Autodesk Fusion 360 part; units mm, degrees
(part 3 of 7)
  line L362 (75.7834, -59.8105) -> (75.8535, -59.6632)
  line L363 (75.8535, -59.6632) -> (76.1212, -59.7821)
  line L364 (76.1212, -59.7821) -> (76.1988, -59.8037)
  line L365 (76.1988, -59.8037) -> (76.2804, -59.8161)
  line L366 (76.2804, -59.8161) -> (76.3647, -59.822)
  line L367 (76.3647, -59.822) -> (76.451, -59.8224)
  line L368 (76.451, -59.8224) -> (76.5391, -59.8175)
  line L369 (76.5391, -59.8175) -> (76.6286, -59.8079)
  line L370 (76.6286, -59.8079) -> (76.7195, -59.7936)
  line L371 (76.7195, -59.7936) -> (76.8114, -59.7747)
  line L372 (76.8114, -59.7747) -> (76.9043, -59.7514)
  line L373 (76.9043, -59.7514) -> (76.9979, -59.7237)
  line L374 (76.9979, -59.7237) -> (77.0921, -59.6916)
  line L375 (77.0921, -59.6916) -> (77.1867, -59.6553)
  line L376 (77.1867, -59.6553) -> (77.2104, -59.5733)
  line L377 (77.2104, -59.5733) -> (77.2325, -59.4909)
  line L378 (77.2325, -59.4909) -> (77.2529, -59.4081)
  line L379 (77.2529, -59.4081) -> (77.1891, -59.3293)
  line L380 (77.1891, -59.3293) -> (77.1236, -59.2545)
  line L381 (77.1236, -59.2545) -> (77.0564, -59.1837)
  line L382 (77.0564, -59.1837) -> (76.9876, -59.117)
  line L383 (76.9876, -59.117) -> (76.9175, -59.0547)
  line L384 (76.9175, -59.0547) -> (76.8459, -58.9969)
  line L385 (76.8459, -58.9969) -> (76.7732, -58.9437)
  line L386 (76.7732, -58.9437) -> (76.6993, -58.8955)
  line L387 (76.6993, -58.8955) -> (76.6244, -58.8526)
  line L388 (76.6244, -58.8526) -> (76.5485, -58.8156)
  line L389 (76.5485, -58.8156) -> (76.4716, -58.7856)
  line L390 (76.4716, -58.7856) -> (76.3936, -58.7655)
  line L391 (76.3936, -58.7655) -> (76.1023, -58.7347)
  line L392 (76.1023, -58.7347) -> (76.1152, -58.572)
  line L393 (76.1152, -58.572) -> (76.1195, -58.4089)
  line L394 (76.1195, -58.4089) -> (76.1152, -58.2458)
  line L395 (76.1152, -58.2458) -> (76.1023, -58.0831)
extrude "Extrude2" add sketch "Sketch2" along normal blind 2.3 separate body makes body 3 in component "CT idler 1"
combine "Combine1" operation add target body 2 tool bodies 3 in component "CT idler 1"
ref_plane "WorkPlane3" through (0, 0, 36.8) normal (0, 0, 1) x (1, 0, 0) in component "CT idler 1"
sketch "Sketch3" plane through (0, 0, 36.8) normal (0, 0, 1) x (1, 0, 0) in component "CT idler 1"
  circle A0 centre (73.0295, -58.4089) radius 2.1
extrude "Extrude3" cut sketch "Sketch3" along normal blind 2 bodies 2 in component "CT idler 1"
ref_plane "WorkPlane4" through (0, 0, 38.8) normal (0, 0, 1) x (1, 0, 0) in component "CT idler 1"
sketch "Sketch4" plane through (0, 0, 38.8) normal (0, 0, 1) x (1, 0, 0) in component "CT idler 1"
  circle A0 centre (73.0295, -58.4089) radius 1.7
extrude "Extrude4" cut sketch "Sketch4" along normal blind 2 bodies 2 in component "CT idler 1"
ref_plane "WorkPlane1" through (0, 0, 39) normal (0, 0, 1) x (1, 0, 0) in component "CT idler 2"
sketch "Sketch1 (3)" plane through (0, 0, 39) normal (0, 0, 1) x (1, 0, 0) in component "CT idler 2"
  line L0 (65.785, -68.2435) -> (66.0567, -68.5986)
  line L1 (66.0567, -68.5986) -> (66.1054, -68.6519)
  line L2 (66.1054, -68.6519) -> (66.1583, -68.702)
  line L3 (66.1583, -68.702) -> (66.2139, -68.7499)
  line L4 (66.2139, -68.7499) -> (66.2719, -68.796)
  line L5 (66.2719, -68.796) -> (66.3318, -68.8405)
  line L6 (66.3318, -68.8405) -> (66.3935, -68.8835)
  line L7 (66.3935, -68.8835) -> (66.457, -68.9251)
  line L8 (66.457, -68.9251) -> (66.522, -68.9654)
  line L9 (66.522, -68.9654) -> (66.5885, -69.0044)
  line L10 (66.5885, -69.0044) -> (66.6564, -69.0422)
  line L11 (66.6564, -69.0422) -> (66.7256, -69.0788)
  line L12 (66.7256, -69.0788) -> (66.7962, -69.1142)
  line L13 (66.7962, -69.1142) -> (66.9045, -69.0248)
  line L14 (66.9045, -69.0248) -> (67.0114, -68.9338)
  line L15 (67.0114, -68.9338) -> (67.117, -68.8411)
  line L16 (67.117, -68.8411) -> (67.0933, -68.7658)
  line L17 (67.0933, -68.7658) -> (67.0683, -68.6916)
  line L18 (67.0683, -68.6916) -> (67.0418, -68.6186)
  line L19 (67.0418, -68.6186) -> (67.014, -68.5467)
  line L20 (67.014, -68.5467) -> (66.9846, -68.4761)
  line L21 (66.9846, -68.4761) -> (66.9536, -68.4068)
  line L22 (66.9536, -68.4068) -> (66.921, -68.339)
  line L23 (66.921, -68.339) -> (66.8867, -68.2727)
  line L24 (66.8867, -68.2727) -> (66.8505, -68.2082)
  line L25 (66.8505, -68.2082) -> (66.8121, -68.1456)
  line L26 (66.8121, -68.1456) -> (66.7711, -68.0854)
  line L27 (66.7711, -68.0854) -> (66.7263, -68.0288)
  line L28 (66.7263, -68.0288) -> (66.4191, -67.7038)
  line L29 (66.4191, -67.7038) -> (66.5706, -67.5567)
  line L30 (66.5706, -67.5567) -> (66.7182, -67.4058)
  line L31 (66.7182, -67.4058) -> (66.8618, -67.251)
  line L32 (66.8618, -67.251) -> (67.0012, -67.0925)
  line L33 (67.0012, -67.0925) -> (67.3409, -67.3834)
  line L34 (67.3409, -67.3834) -> (67.3996, -67.4254)
  line L35 (67.3996, -67.4254) -> (67.4617, -67.4634)
  line L36 (67.4617, -67.4634) -> (67.5261, -67.4986)
  line L37 (67.5261, -67.4986) -> (67.5924, -67.5317)
  line L38 (67.5924, -67.5317) -> (67.6602, -67.5627)
  line L39 (67.6602, -67.5627) -> (67.7296, -67.592)
  line L40 (67.7296, -67.592) -> (67.8003, -67.6195)
  line L41 (67.8003, -67.6195) -> (67.8722, -67.6454)
  line L42 (67.8722, -67.6454) -> (67.9454, -67.6698)
  line L43 (67.9454, -67.6698) -> (68.0197, -67.6926)
  line L44 (68.0197, -67.6926) -> (68.095, -67.714)
  line L45 (68.095, -67.714) -> (68.1714, -67.7339)
  line L46 (68.1714, -67.7339) -> (68.2587, -67.624)
  line L47 (68.2587, -67.624) -> (68.3444, -67.5127)
  line L48 (68.3444, -67.5127) -> (68.4284, -67.4001)
  line L49 (68.4284, -67.4001) -> (68.3896, -67.3314)
  line L50 (68.3896, -67.3314) -> (68.3497, -67.264)
  line L51 (68.3497, -67.264) -> (68.3086, -67.1981)
  line L52 (68.3086, -67.1981) -> (68.2664, -67.1336)
  line L53 (68.2664, -67.1336) -> (68.223, -67.0706)
  line L54 (68.223, -67.0706) -> (68.1783, -67.0093)
  line L55 (68.1783, -67.0093) -> (68.1323, -66.9497)
  line L56 (68.1323, -66.9497) -> (68.085, -66.892)
  line L57 (68.085, -66.892) -> (68.0361, -66.8364)
  line L58 (68.0361, -66.8364) -> (67.9855, -66.7832)
  line L59 (67.9855, -66.7832) -> (67.933, -66.7328)
  line L60 (67.933, -66.7328) -> (67.8774, -66.6868)
  line L61 (67.8774, -66.6868) -> (67.5093, -66.4327)
  line L62 (67.5093, -66.4327) -> (67.627, -66.2574)
  line L63 (67.627, -66.2574) -> (67.74, -66.0791)
  line L64 (67.74, -66.0791) -> (67.8482, -65.8978)
  line L65 (67.8482, -65.8978) -> (67.9516, -65.7137)
  line L66 (67.9516, -65.7137) -> (68.3444, -65.9277)
  line L67 (68.3444, -65.9277) -> (68.4105, -65.9566)
  line L68 (68.4105, -65.9566) -> (68.4792, -65.9808)
  line L69 (68.4792, -65.9808) -> (68.5495, -66.0019)
  line L70 (68.5495, -66.0019) -> (68.6212, -66.0205)
  line L71 (68.6212, -66.0205) -> (68.694, -66.0367)
  line L72 (68.694, -66.0367) -> (68.7679, -66.0509)
  line L73 (68.7679, -66.0509) -> (68.8428, -66.0631)
  line L74 (68.8428, -66.0631) -> (68.9186, -66.0735)
  line L75 (68.9186, -66.0735) -> (68.9952, -66.0821)
  line L76 (68.9952, -66.0821) -> (69.0726, -66.089)
  line L77 (69.0726, -66.089) -> (69.1507, -66.0943)
  line L78 (69.1507, -66.0943) -> (69.2295, -66.0979)
  line L79 (69.2295, -66.0979) -> (69.2921, -65.9722)
  line L80 (69.2921, -65.9722) -> (69.3528, -65.8455)
  line L81 (69.3528, -65.8455) -> (69.4116, -65.718)
  line L82 (69.4116, -65.718) -> (69.3593, -65.6588)
  line L83 (69.3593, -65.6588) -> (69.3063, -65.6012)
  line L84 (69.3063, -65.6012) -> (69.2524, -65.5452)
  line L85 (69.2524, -65.5452) -> (69.1977, -65.4909)
  line L86 (69.1977, -65.4909) -> (69.1421, -65.4383)
  line L87 (69.1421, -65.4383) -> (69.0857, -65.3877)
  line L88 (69.0857, -65.3877) -> (69.0283, -65.3389)
  line L89 (69.0283, -65.3389) -> (68.97, -65.2924)
  line L90 (68.97, -65.2924) -> (68.9106, -65.2481)
  line L91 (68.9106, -65.2481) -> (68.8501, -65.2066)
  line L92 (68.8501, -65.2066) -> (68.7882, -65.1682)
  line L93 (68.7882, -65.1682) -> (68.7243, -65.1348)
  line L94 (68.7243, -65.1348) -> (68.3114, -64.9628)
  line L95 (68.3114, -64.9628) -> (68.3901, -64.7668)
  line L96 (68.3901, -64.7668) -> (68.4635, -64.5689)
  line L97 (68.4635, -64.5689) -> (68.5317, -64.3691)
  line L98 (68.5317, -64.3691) -> (68.5946, -64.1676)
  line L99 (68.5946, -64.1676) -> (69.0232, -64.2952)
  line L100 (69.0232, -64.2952) -> (69.0939, -64.3097)
  line L101 (69.0939, -64.3097) -> (69.1661, -64.3191)
  line L102 (69.1661, -64.3191) -> (69.2393, -64.3251)
  line L103 (69.2393, -64.3251) -> (69.3133, -64.3284)
  line L104 (69.3133, -64.3284) -> (69.3879, -64.3291)
  line L105 (69.3879, -64.3291) -> (69.4631, -64.3276)
  line L106 (69.4631, -64.3276) -> (69.5389, -64.324)
  line L107 (69.5389, -64.324) -> (69.6152, -64.3184)
  line L108 (69.6152, -64.3184) -> (69.6919, -64.3109)
  line L109 (69.6919, -64.3109) -> (69.7691, -64.3016)
  line L110 (69.7691, -64.3016) -> (69.8466, -64.2905)
  line L111 (69.8466, -64.2905) -> (69.9245, -64.2776)
  line L112 (69.9245, -64.2776) -> (69.9595, -64.1416)
  line L113 (69.9595, -64.1416) -> (69.9926, -64.0051)
  line L114 (69.9926, -64.0051) -> (70.0235, -63.8682)
  line L115 (70.0235, -63.8682) -> (69.9601, -63.8211)
  line L116 (69.9601, -63.8211) -> (69.8963, -63.7758)
  line L117 (69.8963, -63.7758) -> (69.8319, -63.7323)
  line L118 (69.8319, -63.7323) -> (69.7671, -63.6905)
  line L119 (69.7671, -63.6905) -> (69.7018, -63.6507)
  line L120 (69.7018, -63.6507) -> (69.6361, -63.6128)
  line L121 (69.6361, -63.6128) -> (69.5698, -63.5771)
  line L122 (69.5698, -63.5771) -> (69.5031, -63.5436)
  line L123 (69.5031, -63.5436) -> (69.4358, -63.5127)
  line L124 (69.4358, -63.5127) -> (69.368, -63.4847)
  line L125 (69.368, -63.4847) -> (69.2995, -63.46)
  line L126 (69.2995, -63.46) -> (69.23, -63.4406)
  line L127 (69.23, -63.4406) -> (68.7904, -63.3582)
  line L128 (68.7904, -63.3582) -> (68.8266, -63.1502)
  line L129 (68.8266, -63.1502) -> (68.8573, -62.9413)
  line L130 (68.8573, -62.9413) -> (68.8824, -62.7317)
  line L131 (68.8824, -62.7317) -> (68.9021, -62.5215)
  line L132 (68.9021, -62.5215) -> (69.3479, -62.5572)
  line L133 (69.3479, -62.5572) -> (69.42, -62.5567)
  line L134 (69.42, -62.5567) -> (69.4926, -62.5509)
  line L135 (69.4926, -62.5509) -> (69.5654, -62.5416)
  line L136 (69.5654, -62.5416) -> (69.6384, -62.5294)
  line L137 (69.6384, -62.5294) -> (69.7116, -62.5146)
  line L138 (69.7116, -62.5146) -> (69.7849, -62.4975)
  line L139 (69.7849, -62.4975) -> (69.8583, -62.4782)
  line L140 (69.8583, -62.4782) -> (69.9317, -62.4569)
  line L141 (69.9317, -62.4569) -> (70.0052, -62.4336)
  line L142 (70.0052, -62.4336) -> (70.0787, -62.4084)
  line L143 (70.0787, -62.4084) -> (70.1522, -62.3814)
  line L144 (70.1522, -62.3814) -> (70.2257, -62.3526)
  line L145 (70.2257, -62.3526) -> (70.2318, -62.2123)
  line L146 (70.2318, -62.2123) -> (70.2357, -62.072)
  line L147 (70.2357, -62.072) -> (70.2375, -61.9315)
  line L148 (70.2375, -61.9315) -> (70.1657, -61.8987)
  line L149 (70.1657, -61.8987) -> (70.0938, -61.8677)
  line L150 (70.0938, -61.8677) -> (70.0218, -61.8384)
  line L151 (70.0218, -61.8384) -> (69.9498, -61.8111)
  line L152 (69.9498, -61.8111) -> (69.8776, -61.7857)
  line L153 (69.8776, -61.7857) -> (69.8054, -61.7623)
  line L154 (69.8054, -61.7623) -> (69.7332, -61.7411)
  line L155 (69.7332, -61.7411) -> (69.661, -61.7223)
  line L156 (69.661, -61.7223) -> (69.5888, -61.706)
  line L157 (69.5888, -61.706) -> (69.5166, -61.6927)
  line L158 (69.5166, -61.6927) -> (69.4444, -61.6829)
  line L159 (69.4444, -61.6829) -> (69.3724, -61.6783)
  line L160 (69.3724, -61.6783) -> (68.9253, -61.6891)
  line L161 (68.9253, -61.6891) -> (68.9174, -61.4781)
  line L162 (68.9174, -61.4781) -> (68.904, -61.2674)
  line L163 (68.904, -61.2674) -> (68.885, -61.0571)
  line L164 (68.885, -61.0571) -> (68.8605, -60.8474)
  line L165 (68.8605, -60.8474) -> (69.304, -60.7897)
  line L166 (69.304, -60.7897) -> (69.3745, -60.7742)
  line L167 (69.3745, -60.7742) -> (69.4443, -60.7534)
  line L168 (69.4443, -60.7534) -> (69.5136, -60.7292)
  line L169 (69.5136, -60.7292) -> (69.5825, -60.7021)
  line L170 (69.5825, -60.7021) -> (69.651, -60.6724)
  line L171 (69.651, -60.6724) -> (69.7191, -60.6404)
  line L172 (69.7191, -60.6404) -> (69.7869, -60.6063)
  line L173 (69.7869, -60.6063) -> (69.8543, -60.5702)
  line L174 (69.8543, -60.5702) -> (69.9213, -60.5321)
  line L175 (69.9213, -60.5321) -> (69.988, -60.4922)
  line L176 (69.988, -60.4922) -> (70.0543, -60.4505)
  line L177 (70.0543, -60.4505) -> (70.1202, -60.4071)
  line L178 (70.1202, -60.4071) -> (70.0969, -60.2686)
  line L179 (70.0969, -60.2686) -> (70.0716, -60.1305)
  line L180 (70.0716, -60.1305) -> (70.0441, -59.9928)
  line L181 (70.0441, -59.9928) -> (69.9671, -59.9756)
  line L182 (69.9671, -59.9756) -> (69.8903, -59.9602)
  line L183 (69.8903, -59.9602) -> (69.8138, -59.9465)
  line L184 (69.8138, -59.9465) -> (69.7377, -59.9347)
  line L185 (69.7377, -59.9347) -> (69.6618, -59.9249)
  line L186 (69.6618, -59.9249) -> (69.5863, -59.9171)
  line L187 (69.5863, -59.9171) -> (69.5113, -59.9114)
  line L188 (69.5113, -59.9114) -> (69.4367, -59.908)
  line L189 (69.4367, -59.908) -> (69.3627, -59.9071)
  line L190 (69.3627, -59.9071) -> (69.2893, -59.909)
  line L191 (69.2893, -59.909) -> (69.2167, -59.9144)
  line L192 (69.2167, -59.9144) -> (69.1453, -59.9249)
  line L193 (69.1453, -59.9249) -> (68.7102, -60.0284)
  line L194 (68.7102, -60.0284) -> (68.6587, -59.8237)
  line L195 (68.6587, -59.8237) -> (68.6017, -59.6204)
  line L196 (68.6017, -59.6204) -> (68.5395, -59.4186)
  line L197 (68.5395, -59.4186) -> (68.4719, -59.2186)
  line L198 (68.4719, -59.2186) -> (68.8937, -59.0699)
  line L199 (68.8937, -59.0699) -> (68.9594, -59.0401)
  line L200 (68.9594, -59.0401) -> (69.0233, -59.0053)
  line L201 (69.0233, -59.0053) -> (69.0861, -58.9672)
  line L202 (69.0861, -58.9672) -> (69.1478, -58.9263)
  line L203 (69.1478, -58.9263) -> (69.2087, -58.8831)
  line L204 (69.2087, -58.8831) -> (69.2687, -58.8376)
  line L205 (69.2687, -58.8376) -> (69.3278, -58.7902)
  line L206 (69.3278, -58.7902) -> (69.3863, -58.7408)
  line L207 (69.3863, -58.7408) -> (69.4439, -58.6896)
  line L208 (69.4439, -58.6896) -> (69.5008, -58.6367)
  line L209 (69.5008, -58.6367) -> (69.557, -58.5822)
  line L210 (69.557, -58.5822) -> (69.6125, -58.526)
  line L211 (69.6125, -58.526) -> (69.5609, -58.3954)
  line L212 (69.5609, -58.3954) -> (69.5074, -58.2655)
  line L213 (69.5074, -58.2655) -> (69.4519, -58.1365)
  line L214 (69.4519, -58.1365) -> (69.373, -58.1357)
  line L215 (69.373, -58.1357) -> (69.2947, -58.1366)
  line L216 (69.2947, -58.1366) -> (69.217, -58.1392)
  line L217 (69.217, -58.1392) -> (69.1401, -58.1435)
  line L218 (69.1401, -58.1435) -> (69.0638, -58.1496)
  line L219 (69.0638, -58.1496) -> (68.9884, -58.1577)
  line L220 (68.9884, -58.1577) -> (68.9138, -58.1677)
  line L221 (68.9138, -58.1677) -> (68.8402, -58.1799)
  line L222 (68.8402, -58.1799) -> (68.7676, -58.1944)
  line L223 (68.7676, -58.1944) -> (68.6962, -58.2115)
  line L224 (68.6962, -58.2115) -> (68.6263, -58.2319)
  line L225 (68.6263, -58.2319) -> (68.5586, -58.2571)
  line L226 (68.5586, -58.2571) -> (68.1546, -58.4487)
  line L227 (68.1546, -58.4487) -> (68.0616, -58.2592)
  line L228 (68.0616, -58.2592) -> (67.9636, -58.0722)
  line L229 (67.9636, -58.0722) -> (67.8608, -57.8878)
  line L230 (67.8608, -57.8878) -> (67.7531, -57.7062)
  line L231 (67.7531, -57.7062) -> (68.1347, -57.4731)
  line L232 (68.1347, -57.4731) -> (68.1928, -57.4302)
  line L233 (68.1928, -57.4302) -> (68.2481, -57.3829)
  line L234 (68.2481, -57.3829) -> (68.3016, -57.3325)
  line L235 (68.3016, -57.3325) -> (68.3535, -57.2797)
  line L236 (68.3535, -57.2797) -> (68.404, -57.2248)
  line L237 (68.404, -57.2248) -> (68.4532, -57.1679)
  line L238 (68.4532, -57.1679) -> (68.5012, -57.1091)
  line L239 (68.5012, -57.1091) -> (68.5481, -57.0487)
  line L240 (68.5481, -57.0487) -> (68.5939, -56.9867)
  line L241 (68.5939, -56.9867) -> (68.6385, -56.9231)
  line L242 (68.6385, -56.9231) -> (68.6822, -56.858)
  line L243 (68.6822, -56.858) -> (68.7247, -56.7916)
  line L244 (68.7247, -56.7916) -> (68.6471, -56.6745)
  line L245 (68.6471, -56.6745) -> (68.5678, -56.5587)
  line L246 (68.5678, -56.5587) -> (68.4867, -56.444)
  line L247 (68.4867, -56.444) -> (68.4094, -56.4596)
  line L248 (68.4094, -56.4596) -> (68.3329, -56.4768)
  line L249 (68.3329, -56.4768) -> (68.2575, -56.4954)
  line L250 (68.2575, -56.4954) -> (68.1831, -56.5157)
  line L251 (68.1831, -56.5157) -> (68.1098, -56.5375)
  line L252 (68.1098, -56.5375) -> (68.0377, -56.561)
  line L253 (68.0377, -56.561) -> (67.9668, -56.5864)
  line L254 (67.9668, -56.5864) -> (67.8973, -56.6136)
  line L255 (67.8973, -56.6136) -> (67.8293, -56.6429)
  line L256 (67.8293, -56.6429) -> (67.7631, -56.6745)
  line L257 (67.7631, -56.6745) -> (67.6989, -56.709)
  line L258 (67.6989, -56.709) -> (67.638, -56.7476)
  line L259 (67.638, -56.7476) -> (67.2826, -57.0191)
  line L260 (67.2826, -57.0191) -> (67.1522, -56.8531)
  line L261 (67.1522, -56.8531) -> (67.0175, -56.6905)
  line L262 (67.0175, -56.6905) -> (66.8786, -56.5315)
  line L263 (66.8786, -56.5315) -> (66.7355, -56.3763)
  line L264 (66.7355, -56.3763) -> (67.0604, -56.0689)
  line L265 (67.0604, -56.0689) -> (67.1083, -56.0149)
  line L266 (67.1083, -56.0149) -> (67.1525, -55.9571)
  line L267 (67.1525, -55.9571) -> (67.1943, -55.8967)
  line L268 (67.1943, -55.8967) -> (67.2341, -55.8343)
  line L269 (67.2341, -55.8343) -> (67.2721, -55.7701)
  line L270 (67.2721, -55.7701) -> (67.3084, -55.7041)
  line L271 (67.3084, -55.7041) -> (67.3432, -55.6367)
  line L272 (67.3432, -55.6367) -> (67.3765, -55.5679)
  line L273 (67.3765, -55.5679) -> (67.4083, -55.4977)
  line L274 (67.4083, -55.4977) -> (67.4388, -55.4262)
  line L275 (67.4388, -55.4262) -> (67.468, -55.3535)
  line L276 (67.468, -55.3535) -> (67.4958, -55.2796)
  line L277 (67.4958, -55.2796) -> (67.3955, -55.1813)
  line L278 (67.3955, -55.1813) -> (67.2938, -55.0844)
  line L279 (67.2938, -55.0844) -> (67.1907, -54.9891)
  line L280 (67.1907, -54.9891) -> (67.1183, -55.0205)
  line L281 (67.1183, -55.0205) -> (67.0471, -55.0532)
  line L282 (67.0471, -55.0532) -> (66.9772, -55.0871)
  line L283 (66.9772, -55.0871) -> (66.9086, -55.1223)
  line L284 (66.9086, -55.1223) -> (66.8415, -55.1589)
  line L285 (66.8415, -55.1589) -> (66.7758, -55.197)
  line L286 (66.7758, -55.197) -> (66.7118, -55.2365)
  line L287 (66.7118, -55.2365) -> (66.6495, -55.2775)
  line L288 (66.6495, -55.2775) -> (66.589, -55.3203)
  line L289 (66.589, -55.3203) -> (66.5308, -55.365)
  line L290 (66.5308, -55.365) -> (66.4752, -55.4121)
  line L291 (66.4752, -55.4121) -> (66.4237, -55.4626)
  line L292 (66.4237, -55.4626) -> (66.1325, -55.802)
  line L293 (66.1325, -55.802) -> (65.9704, -55.6667)
  line L294 (65.9704, -55.6667) -> (65.8049, -55.5357)
  line L295 (65.8049, -55.5357) -> (65.6359, -55.4091)
  line L296 (65.6359, -55.4091) -> (65.4637, -55.287)
  line L297 (65.4637, -55.287) -> (65.7175, -54.9188)
  line L298 (65.7175, -54.9188) -> (65.7532, -54.856)
  line L299 (65.7532, -54.856) -> (65.7844, -54.7903)
  line L300 (65.7844, -54.7903) -> (65.8128, -54.7225)
  line L301 (65.8128, -54.7225) -> (65.8387, -54.6532)
  line L302 (65.8387, -54.6532) -> (65.8625, -54.5824)
  line L303 (65.8625, -54.5824) -> (65.8844, -54.5104)
  line L304 (65.8844, -54.5104) -> (65.9043, -54.4372)
  line L305 (65.9043, -54.4372) -> (65.9226, -54.363)
  line L306 (65.9226, -54.363) -> (65.9391, -54.2877)
  line L307 (65.9391, -54.2877) -> (65.9541, -54.2114)
  line L308 (65.9541, -54.2114) -> (65.9675, -54.1343)
  line L309 (65.9675, -54.1343) -> (65.9793, -54.0562)
  line L310 (65.9793, -54.0562) -> (65.8608, -53.9809)
  line L311 (65.8608, -53.9809) -> (65.7412, -53.9073)
  line L312 (65.7412, -53.9073) -> (65.6205, -53.8355)
  line L313 (65.6205, -53.8355) -> (65.5562, -53.8813)
  line L314 (65.5562, -53.8813) -> (65.4934, -53.928)
  line L315 (65.4934, -53.928) -> (65.4321, -53.9757)
  line L316 (65.4321, -53.9757) -> (65.3723, -54.0244)
  line L317 (65.3723, -54.0244) -> (65.3143, -54.0742)
  line L318 (65.3143, -54.0742) -> (65.2579, -54.1251)
  line L319 (65.2579, -54.1251) -> (65.2035, -54.177)
  line L320 (65.2035, -54.177) -> (65.1511, -54.2301)
  line L321 (65.1511, -54.2301) -> (65.1009, -54.2846)
  line L322 (65.1009, -54.2846) -> (65.0532, -54.3404)
  line L323 (65.0532, -54.3404) -> (65.0086, -54.398)
  line L324 (65.0086, -54.398) -> (64.9687, -54.4581)
  line L325 (64.9687, -54.4581) -> (64.7545, -54.8507)
  line L326 (64.7545, -54.8507) -> (64.5678, -54.752)
  line L327 (64.5678, -54.752) -> (64.3786, -54.6583)
  line L328 (64.3786, -54.6583) -> (64.187, -54.5695)
  line L329 (64.187, -54.5695) -> (63.9932, -54.4859)
  line L330 (63.9932, -54.4859) -> (64.1649, -54.073)
  line L331 (64.1649, -54.073) -> (64.1867, -54.0042)
  line L332 (64.1867, -54.0042) -> (64.2036, -53.9334)
  line L333 (64.2036, -53.9334) -> (64.2173, -53.8612)
  line L334 (64.2173, -53.8612) -> (64.2283, -53.788)
  line L335 (64.2283, -53.788) -> (64.2368, -53.7139)
  line L336 (64.2368, -53.7139) -> (64.2432, -53.6389)
  line L337 (64.2432, -53.6389) -> (64.2475, -53.5631)
  line L338 (64.2475, -53.5631) -> (64.2499, -53.4867)
  line L339 (64.2499, -53.4867) -> (64.2505, -53.4096)
  line L340 (64.2505, -53.4096) -> (64.2492, -53.3319)
  line L341 (64.2492, -53.3319) -> (64.2463, -53.2536)
  line L342 (64.2463, -53.2536) -> (64.2417, -53.1749)
  line L343 (64.2417, -53.1749) -> (64.1101, -53.1258)
  line L344 (64.1101, -53.1258) -> (63.9778, -53.0786)
  line L345 (63.9778, -53.0786) -> (63.8448, -53.0335)
  line L346 (63.8448, -53.0335) -> (63.7914, -53.0917)
  line L347 (63.7914, -53.0917) -> (63.7397, -53.1504)
  line L348 (63.7397, -53.1504) -> (63.6896, -53.2099)
  line L349 (63.6896, -53.2099) -> (63.6413, -53.27)
  line L350 (63.6413, -53.27) -> (63.5949, -53.3307)
  line L351 (63.5949, -53.3307) -> (63.5503, -53.3922)
  line L352 (63.5503, -53.3922) -> (63.5079, -53.4543)
  line L353 (63.5079, -53.4543) -> (63.4677, -53.5172)
  line L354 (63.4677, -53.5172) -> (63.4299, -53.5808)
  line L355 (63.4299, -53.5808) -> (63.3949, -53.6454)
  line L356 (63.3949, -53.6454) -> (63.3632, -53.7109)
  line L357 (63.3632, -53.7109) -> (63.3367, -53.778)
  line L358 (63.3367, -53.778) -> (63.2087, -54.2066)
  line L359 (63.2087, -54.2066) -> (63.0056, -54.1489)
  line L360 (63.0056, -54.1489) -> (62.8011, -54.0965)
  line L361 (62.8011, -54.0965) -> (62.5953, -54.0496)
  line L362 (62.5953, -54.0496) -> (62.3883, -54.0081)
  line L363 (62.3883, -54.0081) -> (62.4704, -53.5685)
  line L364 (62.4704, -53.5685) -> (62.4774, -53.4966)
  line L365 (62.4774, -53.4966) -> (62.4792, -53.4239)
  line L366 (62.4792, -53.4239) -> (62.4776, -53.3505)
  line L367 (62.4776, -53.3505) -> (62.4731, -53.2766)
  line L368 (62.4731, -53.2766) -> (62.466, -53.2022)
  line L369 (62.466, -53.2022) -> (62.4567, -53.1276)
  line L370 (62.4567, -53.1276) -> (62.4452, -53.0526)
  line L371 (62.4452, -53.0526) -> (62.4316, -52.9773)
  line L372 (62.4316, -52.9773) -> (62.4161, -52.9018)
  line L373 (62.4161, -52.9018) -> (62.3988, -52.8261)
  line L374 (62.3988, -52.8261) -> (62.3796, -52.7501)
  line L375 (62.3796, -52.7501) -> (62.3587, -52.674)
  line L376 (62.3587, -52.674) -> (62.2198, -52.6533)
  line L377 (62.2198, -52.6533) -> (62.0806, -52.6348)
  line L378 (62.0806, -52.6348) -> (61.9412, -52.6183)
  line L379 (61.9412, -52.6183) -> (61.901, -52.6863)
  line L380 (61.901, -52.6863) -> (61.8626, -52.7545)
  line L381 (61.8626, -52.7545) -> (61.826, -52.8231)
  line L382 (61.826, -52.8231) -> (61.7913, -52.8919)
  line L383 (61.7913, -52.8919) -> (61.7585, -52.961)
  line L384 (61.7585, -52.961) -> (61.7277, -53.0303)
  line L385 (61.7277, -53.0303) -> (61.6991, -53.0999)
  line L386 (61.6991, -53.0999) -> (61.6728, -53.1698)
  line L387 (61.6728, -53.1698) -> (61.6491, -53.2399)
  line L388 (61.6491, -53.2399) -> (61.6283, -53.3103)
  line L389 (61.6283, -53.3103) -> (61.6109, -53.381)
  line L390 (61.6109, -53.381) -> (61.5989, -53.4522)
  line L391 (61.5989, -53.4522) -> (61.5629, -53.898)
  line L392 (61.5629, -53.898) -> (61.3522, -53.8837)
  line L393 (61.3522, -53.8837) -> (61.1413, -53.8751)
  line L394 (61.1413, -53.8751) -> (60.9302, -53.8719)
  line L395 (60.9302, -53.8719) -> (60.7191, -53.8744)
  line L396 (60.7191, -53.8744) -> (60.708, -53.4273)
  line L397 (60.708, -53.4273) -> (60.6999, -53.3556)
  line L398 (60.6999, -53.3556) -> (60.6866, -53.284)
  line L399 (60.6866, -53.284) -> (60.6697, -53.2125)
  line L400 (60.6697, -53.2125) -> (60.6499, -53.1412)
  line L401 (60.6499, -53.1412) -> (60.6276, -53.07)
  line L402 (60.6276, -53.07) -> (60.6029, -52.9989)
  line L403 (60.6029, -52.9989) -> (60.5761, -52.9279)
  line L404 (60.5761, -52.9279) -> (60.5472, -52.8571)
  line L405 (60.5472, -52.8571) -> (60.5163, -52.7865)
  line L406 (60.5163, -52.7865) -> (60.4836, -52.716)
  line L407 (60.4836, -52.716) -> (60.4491, -52.6457)
  line L408 (60.4491, -52.6457) -> (60.4128, -52.5756)
  line L409 (60.4128, -52.5756) -> (60.2726, -52.5843)
  line L410 (60.2726, -52.5843) -> (60.1326, -52.595)
  line L411 (60.1326, -52.595) -> (59.9928, -52.6079)
  line L412 (59.9928, -52.6079) -> (59.9676, -52.6827)
  line L413 (59.9676, -52.6827) -> (59.9443, -52.7575)
  line L414 (59.9443, -52.7575) -> (59.9227, -52.8321)
  line L415 (59.9227, -52.8321) -> (59.903, -52.9067)
  line L416 (59.903, -52.9067) -> (59.8853, -52.9811)
  line L417 (59.8853, -52.9811) -> (59.8696, -53.0553)
  line L418 (59.8696, -53.0553) -> (59.8561, -53.1293)
  line L419 (59.8561, -53.1293) -> (59.8449, -53.2031)
  line L420 (59.8449, -53.2031) -> (59.8363, -53.2767)
  line L421 (59.8363, -53.2767) -> (59.8306, -53.3499)
  line L422 (59.8306, -53.3499) -> (59.8284, -53.4226)
  line L423 (59.8284, -53.4226) -> (59.8314, -53.4947)
  line L424 (59.8314, -53.4947) -> (59.8888, -53.9383)
  line L425 (59.8888, -53.9383) -> (59.6798, -53.9682)
  line L426 (59.6798, -53.9682) -> (59.4717, -54.0035)
  line L427 (59.4717, -54.0035) -> (59.2645, -54.0444)
  line L428 (59.2645, -54.0444) -> (59.0585, -54.0907)
  line L429 (59.0585, -54.0907) -> (58.9547, -53.6556)
  line L430 (58.9547, -53.6556) -> (58.9319, -53.5872)
  line L431 (58.9319, -53.5872) -> (58.904, -53.5199)
  line L432 (58.904, -53.5199) -> (58.8727, -53.4535)
  line L433 (58.8727, -53.4535) -> (58.8385, -53.3879)
  line L434 (58.8385, -53.3879) -> (58.8018, -53.3228)
  line L435 (58.8018, -53.3228) -> (58.7629, -53.2584)
  line L436 (58.7629, -53.2584) -> (58.7219, -53.1946)
  line L437 (58.7219, -53.1946) -> (58.6789, -53.1314)
  line L438 (58.6789, -53.1314) -> (58.634, -53.0687)
  line L439 (58.634, -53.0687) -> (58.5874, -53.0065)
  line L440 (58.5874, -53.0065) -> (58.539, -52.945)
  line L441 (58.539, -52.945) -> (58.4889, -52.8839)
  line L442 (58.4889, -52.8839) -> (58.3536, -52.9216)
  line L443 (58.3536, -52.9216) -> (58.2189, -52.9612)
  line L444 (58.2189, -52.9612) -> (58.0848, -53.0029)
  line L445 (58.0848, -53.0029) -> (58.0758, -53.0813)
  line L446 (58.0758, -53.0813) -> (58.0685, -53.1593)
  line L447 (58.0685, -53.1593) -> (58.0629, -53.2368)
  line L448 (58.0629, -53.2368) -> (58.0592, -53.3138)
  line L449 (58.0592, -53.3138) -> (58.0573, -53.3902)
  line L450 (58.0573, -53.3902) -> (58.0574, -53.4661)
  line L451 (58.0574, -53.4661) -> (58.0596, -53.5413)
  line L452 (58.0596, -53.5413) -> (58.064, -53.6158)
  line L453 (58.064, -53.6158) -> (58.0708, -53.6895)
  line L454 (58.0708, -53.6895) -> (58.0804, -53.7623)
  line L455 (58.0804, -53.7623) -> (58.0934, -53.834)
  line L456 (58.0934, -53.834) -> (58.1113, -53.9039)
  line L457 (58.1113, -53.9039) -> (58.2597, -54.3258)
  line L458 (58.2597, -54.3258) -> (58.0615, -54.3984)
  line L459 (58.0615, -54.3984) -> (57.8652, -54.4763)
  line L460 (57.8652, -54.4763) -> (57.6711, -54.5593)
  line L461 (57.6711, -54.5593) -> (57.4793, -54.6474)
  line L462 (57.4793, -54.6474) -> (57.2873, -54.2435)
  line L463 (57.2873, -54.2435) -> (57.2508, -54.1813)
  line L464 (57.2508, -54.1813) -> (57.2095, -54.1213)
  line L465 (57.2095, -54.1213) -> (57.165, -54.0629)
  line L466 (57.165, -54.0629) -> (57.1179, -54.0058)
  line L467 (57.1179, -54.0058) -> (57.0685, -53.9498)
  line L468 (57.0685, -53.9498) -> (57.0171, -53.8949)
  line L469 (57.0171, -53.8949) -> (56.9637, -53.841)
  line L470 (56.9637, -53.841) -> (56.9085, -53.788)
  line L471 (56.9085, -53.788) -> (56.8516, -53.736)
  line L472 (56.8516, -53.736) -> (56.793, -53.685)
  line L473 (56.793, -53.685) -> (56.7329, -53.6348)
  line L474 (56.7329, -53.6348) -> (56.6712, -53.5855)
  line L475 (56.6712, -53.5855) -> (56.5467, -53.6504)
  line L476 (56.5467, -53.6504) -> (56.4232, -53.7172)
  line L477 (56.4232, -53.7172) -> (56.3007, -53.7859)
  line L478 (56.3007, -53.7859) -> (56.3081, -53.8645)
  line L479 (56.3081, -53.8645) -> (56.3172, -53.9422)
  line L480 (56.3172, -53.9422) -> (56.3279, -54.0192)
  line L481 (56.3279, -54.0192) -> (56.3402, -54.0953)
  line L482 (56.3402, -54.0953) -> (56.3543, -54.1705)
  line L483 (56.3543, -54.1705) -> (56.3701, -54.2447)
  line L484 (56.3701, -54.2447) -> (56.3879, -54.3178)
  line L485 (56.3879, -54.3178) -> (56.4077, -54.3898)
  line L486 (56.4077, -54.3898) -> (56.4297, -54.4604)
  line L487 (56.4297, -54.4604) -> (56.4543, -54.5296)
  line L488 (56.4543, -54.5296) -> (56.4818, -54.597)
  line L489 (56.4818, -54.597) -> (56.5139, -54.6617)
  line L490 (56.5139, -54.6617) -> (56.7468, -55.0435)
  line L491 (56.7468, -55.0435) -> (56.568, -55.1558)
  line L492 (56.568, -55.1558) -> (56.3922, -55.2728)
  line L493 (56.3922, -55.2728) -> (56.2196, -55.3943)
  line L494 (56.2196, -55.3943) -> (56.0503, -55.5204)
  line L495 (56.0503, -55.5204) -> (55.7785, -55.1652)
  line L496 (55.7785, -55.1652) -> (55.7298, -55.1119)
  line L497 (55.7298, -55.1119) -> (55.677, -55.0619)
  line L498 (55.677, -55.0619) -> (55.6213, -55.014)
  line L499 (55.6213, -55.014) -> (55.5634, -54.9679)
  line L500 (55.5634, -54.9679) -> (55.5035, -54.9234)
  line L501 (55.5035, -54.9234) -> (55.4417, -54.8804)
  line L502 (55.4417, -54.8804) -> (55.3783, -54.8387)
  line L503 (55.3783, -54.8387) -> (55.3133, -54.7984)
  line L504 (55.3133, -54.7984) -> (55.2468, -54.7594)
  line L505 (55.2468, -54.7594) -> (55.1789, -54.7216)
  line L506 (55.1789, -54.7216) -> (55.1096, -54.6851)
  line L507 (55.1096, -54.6851) -> (55.0391, -54.6497)
  line L508 (55.0391, -54.6497) -> (54.9308, -54.7391)
  line L509 (54.9308, -54.7391) -> (54.8238, -54.8301)
  line L510 (54.8238, -54.8301) -> (54.7183, -54.9227)
  line L511 (54.7183, -54.9227) -> (54.7419, -54.998)
  line L512 (54.7419, -54.998) -> (54.767, -55.0722)
  line L513 (54.767, -55.0722) -> (54.7934, -55.1453)
  line L514 (54.7934, -55.1453) -> (54.8213, -55.2172)
  line L515 (54.8213, -55.2172) -> (54.8507, -55.2878)
  line L516 (54.8507, -55.2878) -> (54.8816, -55.357)
  line L517 (54.8816, -55.357) -> (54.9142, -55.4249)
  line L518 (54.9142, -55.4249) -> (54.9486, -55.4911)
  line L519 (54.9486, -55.4911) -> (54.9848, -55.5557)
  line L520 (54.9848, -55.5557) -> (55.0232, -55.6183)
  line L521 (55.0232, -55.6183) -> (55.0641, -55.6785)
  line L522 (55.0641, -55.6785) -> (55.109, -55.735)
  line L523 (55.109, -55.735) -> (55.4161, -56.0601)
  line L524 (55.4161, -56.0601) -> (55.2646, -56.2071)
  line L525 (55.2646, -56.2071) -> (55.117, -56.3581)
  line L526 (55.117, -56.3581) -> (54.9734, -56.5129)
  line L527 (54.9734, -56.5129) -> (54.834, -56.6714)
  line L528 (54.834, -56.6714) -> (54.4943, -56.3805)
  line L529 (54.4943, -56.3805) -> (54.4356, -56.3385)
  line L530 (54.4356, -56.3385) -> (54.3735, -56.3005)
  line L531 (54.3735, -56.3005) -> (54.3091, -56.2652)
  line L532 (54.3091, -56.2652) -> (54.2429, -56.2322)
  line L533 (54.2429, -56.2322) -> (54.175, -56.2011)
  line L534 (54.175, -56.2011) -> (54.1057, -56.1719)
  line L535 (54.1057, -56.1719) -> (54.035, -56.1444)
  line L536 (54.035, -56.1444) -> (53.963, -56.1184)
  line L537 (53.963, -56.1184) -> (53.8899, -56.0941)
  line L538 (53.8899, -56.0941) -> (53.8156, -56.0713)
  line L539 (53.8156, -56.0713) -> (53.7402, -56.0499)
  line L540 (53.7402, -56.0499) -> (53.6639, -56.0299)
  line L541 (53.6639, -56.0299) -> (53.5765, -56.1399)
  line L542 (53.5765, -56.1399) -> (53.4909, -56.2512)
  line L543 (53.4909, -56.2512) -> (53.4069, -56.3637)
  line L544 (53.4069, -56.3637) -> (53.4456, -56.4324)
  line L545 (53.4456, -56.4324) -> (53.4855, -56.4998)
  line L546 (53.4855, -56.4998) -> (53.5266, -56.5658)
  line L547 (53.5266, -56.5658) -> (53.5688, -56.6303)
  line L548 (53.5688, -56.6303) -> (53.6123, -56.6933)
  line L549 (53.6123, -56.6933) -> (53.6569, -56.7546)
  line L550 (53.6569, -56.7546) -> (53.7029, -56.8142)
  line L551 (53.7029, -56.8142) -> (53.7503, -56.8718)
  line L552 (53.7503, -56.8718) -> (53.7991, -56.9275)
  line L553 (53.7991, -56.9275) -> (53.8497, -56.9807)
  line L554 (53.8497, -56.9807) -> (53.9023, -57.031)
  line L555 (53.9023, -57.031) -> (53.9579, -57.0771)
  line L556 (53.9579, -57.0771) -> (54.3259, -57.3311)
  line L557 (54.3259, -57.3311) -> (54.2083, -57.5065)
  line L558 (54.2083, -57.5065) -> (54.0953, -57.6848)
  line L559 (54.0953, -57.6848) -> (53.987, -57.8661)
  line L560 (53.987, -57.8661) -> (53.8836, -58.0501)
  line L561 (53.8836, -58.0501) -> (53.4909, -57.8362)
  line L562 (53.4909, -57.8362) -> (53.4247, -57.8073)
  line L563 (53.4247, -57.8073) -> (53.3561, -57.7831)
  line L564 (53.3561, -57.7831) -> (53.2858, -57.7619)
  line L565 (53.2858, -57.7619) -> (53.2141, -57.7434)
  line L566 (53.2141, -57.7434) -> (53.1412, -57.7271)
  line L567 (53.1412, -57.7271) -> (53.0673, -57.7129)
  line L568 (53.0673, -57.7129) -> (52.9925, -57.7007)
  line L569 (52.9925, -57.7007) -> (52.9167, -57.6903)
  line L570 (52.9167, -57.6903) -> (52.8401, -57.6817)
  line L571 (52.8401, -57.6817) -> (52.7627, -57.6748)
  line L572 (52.7627, -57.6748) -> (52.6845, -57.6696)
  line L573 (52.6845, -57.6696) -> (52.6057, -57.666)
  line L574 (52.6057, -57.666) -> (52.5431, -57.7917)
  line L575 (52.5431, -57.7917) -> (52.4824, -57.9183)
  line L576 (52.4824, -57.9183) -> (52.4237, -58.0459)
  line L577 (52.4237, -58.0459) -> (52.4759, -58.105)
  line L578 (52.4759, -58.105) -> (52.529, -58.1627)
  line L579 (52.529, -58.1627) -> (52.5828, -58.2187)
  line L580 (52.5828, -58.2187) -> (52.6375, -58.273)
  line L581 (52.6375, -58.273) -> (52.6931, -58.3255)
  line L582 (52.6931, -58.3255) -> (52.7496, -58.3762)
  line L583 (52.7496, -58.3762) -> (52.8069, -58.4249)
  line L584 (52.8069, -58.4249) -> (52.8652, -58.4715)
  line L585 (52.8652, -58.4715) -> (52.9246, -58.5157)
  line L586 (52.9246, -58.5157) -> (52.9851, -58.5573)
  line L587 (52.9851, -58.5573) -> (53.047, -58.5956)
  line L588 (53.047, -58.5956) -> (53.111, -58.6291)
  line L589 (53.111, -58.6291) -> (53.5238, -58.8011)
  line L590 (53.5238, -58.8011) -> (53.4452, -58.997)
  line L591 (53.4452, -58.997) -> (53.3717, -59.195)
  line L592 (53.3717, -59.195) -> (53.3035, -59.3948)
  line L593 (53.3035, -59.3948) -> (53.2406, -59.5963)
  line L594 (53.2406, -59.5963) -> (52.812, -59.4687)
  line L595 (52.812, -59.4687) -> (52.7413, -59.4542)
  line L596 (52.7413, -59.4542) -> (52.6691, -59.4448)
  line L597 (52.6691, -59.4448) -> (52.5959, -59.4387)
  line L598 (52.5959, -59.4387) -> (52.522, -59.4355)
  line L599 (52.522, -59.4355) -> (52.4473, -59.4347)
  line L600 (52.4473, -59.4347) -> (52.3721, -59.4362)
  line L601 (52.3721, -59.4362) -> (52.2963, -59.4398)
  line L602 (52.2963, -59.4398) -> (52.22, -59.4454)
  line L603 (52.22, -59.4454) -> (52.1433, -59.4529)
  line L604 (52.1433, -59.4529) -> (52.0662, -59.4623)
  line L605 (52.0662, -59.4623) -> (51.9887, -59.4734)
  line L606 (51.9887, -59.4734) -> (51.9108, -59.4862)
  line L607 (51.9108, -59.4862) -> (51.8757, -59.6222)
  line L608 (51.8757, -59.6222) -> (51.8427, -59.7587)
  line L609 (51.8427, -59.7587) -> (51.8117, -59.8957)
  line L610 (51.8117, -59.8957) -> (51.8751, -59.9427)
  line L611 (51.8751, -59.9427) -> (51.939, -59.988)
  line L612 (51.939, -59.988) -> (52.0033, -60.0316)
  line L613 (52.0033, -60.0316) -> (52.0681, -60.0734)
  line L614 (52.0681, -60.0734) -> (52.1334, -60.1132)
  line L615 (52.1334, -60.1132) -> (52.1992, -60.151)
  line L616 (52.1992, -60.151) -> (52.2654, -60.1868)
  line L617 (52.2654, -60.1868) -> (52.3321, -60.2202)
  line L618 (52.3321, -60.2202) -> (52.3994, -60.2511)
  line L619 (52.3994, -60.2511) -> (52.4672, -60.2792)
  line L620 (52.4672, -60.2792) -> (52.5358, -60.3038)
  line L621 (52.5358, -60.3038) -> (52.6053, -60.3232)
  line L622 (52.6053, -60.3232) -> (53.0448, -60.4057)
  line L623 (53.0448, -60.4057) -> (53.0087, -60.6137)
  line L624 (53.0087, -60.6137) -> (52.978, -60.8226)
  line L625 (52.978, -60.8226) -> (52.9528, -61.0322)
  line L626 (52.9528, -61.0322) -> (52.9332, -61.2424)
  line L627 (52.9332, -61.2424) -> (52.4874, -61.2067)
  line L628 (52.4874, -61.2067) -> (52.4152, -61.2072)
  line L629 (52.4152, -61.2072) -> (52.3426, -61.213)
  line L630 (52.3426, -61.213) -> (52.2698, -61.2223)
  line L631 (52.2698, -61.2223) -> (52.1968, -61.2345)
  line L632 (52.1968, -61.2345) -> (52.1236, -61.2493)
  line L633 (52.1236, -61.2493) -> (52.0503, -61.2664)
  line L634 (52.0503, -61.2664) -> (51.977, -61.2857)
  line L635 (51.977, -61.2857) -> (51.9035, -61.307)
  line L636 (51.9035, -61.307) -> (51.83, -61.3303)
  line L637 (51.83, -61.3303) -> (51.7565, -61.3555)
  line L638 (51.7565, -61.3555) -> (51.683, -61.3825)
  line L639 (51.683, -61.3825) -> (51.6095, -61.4112)
  line L640 (51.6095, -61.4112) -> (51.6035, -61.5515)
  line L641 (51.6035, -61.5515) -> (51.5996, -61.6919)
  line L642 (51.5996, -61.6919) -> (51.5978, -61.8323)
  line L643 (51.5978, -61.8323) -> (51.6695, -61.8651)
  line L644 (51.6695, -61.8651) -> (51.7414, -61.8962)
  line L645 (51.7414, -61.8962) -> (51.8134, -61.9254)
  line L646 (51.8134, -61.9254) -> (51.8855, -61.9528)
  line L647 (51.8855, -61.9528) -> (51.9576, -61.9782)
  line L648 (51.9576, -61.9782) -> (52.0298, -62.0015)
  line L649 (52.0298, -62.0015) -> (52.102, -62.0227)
  line L650 (52.102, -62.0227) -> (52.1743, -62.0415)
  line L651 (52.1743, -62.0415) -> (52.2465, -62.0578)
  line L652 (52.2465, -62.0578) -> (52.3187, -62.0712)
  line L653 (52.3187, -62.0712) -> (52.3908, -62.081)
  line L654 (52.3908, -62.081) -> (52.4628, -62.0855)
  line L655 (52.4628, -62.0855) -> (52.9099, -62.0748)
  line L656 (52.9099, -62.0748) -> (52.9178, -62.2858)
  line L657 (52.9178, -62.2858) -> (52.9312, -62.4964)
  line L658 (52.9312, -62.4964) -> (52.9502, -62.7067)
  line L659 (52.9502, -62.7067) -> (52.9747, -62.9164)
  line L660 (52.9747, -62.9164) -> (52.5312, -62.9742)
  line L661 (52.5312, -62.9742) -> (52.4607, -62.9897)
  line L662 (52.4607, -62.9897) -> (52.391, -63.0104)
  line L663 (52.391, -63.0104) -> (52.3216, -63.0347)
  line L664 (52.3216, -63.0347) -> (52.2528, -63.0618)
  line L665 (52.2528, -63.0618) -> (52.1843, -63.0915)
  line L666 (52.1843, -63.0915) -> (52.1161, -63.1234)
  line L667 (52.1161, -63.1234) -> (52.0484, -63.1576)
  line L668 (52.0484, -63.1576) -> (51.981, -63.1937)
  line L669 (51.981, -63.1937) -> (51.9139, -63.2318)
  line L670 (51.9139, -63.2318) -> (51.8473, -63.2717)
  line L671 (51.8473, -63.2717) -> (51.781, -63.3134)
  line L672 (51.781, -63.3134) -> (51.7151, -63.3568)
  line L673 (51.7151, -63.3568) -> (51.7383, -63.4953)
  line L674 (51.7383, -63.4953) -> (51.7637, -63.6334)
  line L675 (51.7637, -63.6334) -> (51.7911, -63.7711)
  line L676 (51.7911, -63.7711) -> (51.8681, -63.7883)
  line L677 (51.8681, -63.7883) -> (51.9449, -63.8037)
  line L678 (51.9449, -63.8037) -> (52.0214, -63.8173)
  line L679 (52.0214, -63.8173) -> (52.0976, -63.8291)
  line L680 (52.0976, -63.8291) -> (52.1734, -63.839)
  line L681 (52.1734, -63.839) -> (52.2489, -63.8468)
  line L682 (52.2489, -63.8468) -> (52.3239, -63.8525)
  line L683 (52.3239, -63.8525) -> (52.3985, -63.8559)
  line L684 (52.3985, -63.8559) -> (52.4725, -63.8568)
  line L685 (52.4725, -63.8568) -> (52.5459, -63.8549)
  line L686 (52.5459, -63.8549) -> (52.6185, -63.8495)
  line L687 (52.6185, -63.8495) -> (52.6899, -63.8389)
  line L688 (52.6899, -63.8389) -> (53.125, -63.7354)
  line L689 (53.125, -63.7354) -> (53.1766, -63.9402)
  line L690 (53.1766, -63.9402) -> (53.2335, -64.1435)
  line L691 (53.2335, -64.1435) -> (53.2958, -64.3452)
  line L692 (53.2958, -64.3452) -> (53.3634, -64.5452)
  line L693 (53.3634, -64.5452) -> (52.9416, -64.6939)
  line L694 (52.9416, -64.6939) -> (52.8759, -64.7238)
  line L695 (52.8759, -64.7238) -> (52.8119, -64.7586)
  line L696 (52.8119, -64.7586) -> (52.7492, -64.7967)
  line L697 (52.7492, -64.7967) -> (52.6874, -64.8375)
  line L698 (52.6874, -64.8375) -> (52.6266, -64.8808)
  line L699 (52.6266, -64.8808) -> (52.5666, -64.9262)
  line L700 (52.5666, -64.9262) -> (52.5074, -64.9737)
  line L701 (52.5074, -64.9737) -> (52.449, -65.0231)
  line L702 (52.449, -65.0231) -> (52.3913, -65.0742)
  line L703 (52.3913, -65.0742) -> (52.3344, -65.1271)
  line L704 (52.3344, -65.1271) -> (52.2782, -65.1817)
  line L705 (52.2782, -65.1817) -> (52.2228, -65.2379)
  line L706 (52.2228, -65.2379) -> (52.2743, -65.3685)
  line L707 (52.2743, -65.3685) -> (52.3279, -65.4983)
  line L708 (52.3279, -65.4983) -> (52.3833, -65.6273)
  line L709 (52.3833, -65.6273) -> (52.4622, -65.6281)
  line L710 (52.4622, -65.6281) -> (52.5405, -65.6272)
  line L711 (52.5405, -65.6272) -> (52.6182, -65.6247)
  line L712 (52.6182, -65.6247) -> (52.6952, -65.6204)
  line L713 (52.6952, -65.6204) -> (52.7714, -65.6142)
  line L714 (52.7714, -65.6142) -> (52.8469, -65.6062)
  line L715 (52.8469, -65.6062) -> (52.9214, -65.5962)
  line L716 (52.9214, -65.5962) -> (52.9951, -65.584)
  line L717 (52.9951, -65.584) -> (53.0677, -65.5695)
  line L718 (53.0677, -65.5695) -> (53.1391, -65.5523)
  line L719 (53.1391, -65.5523) -> (53.209, -65.5319)
  line L720 (53.209, -65.5319) -> (53.2766, -65.5068)
  line L721 (53.2766, -65.5068) -> (53.6807, -65.3151)
  line L722 (53.6807, -65.3151) -> (53.7737, -65.5047)
  line L723 (53.7737, -65.5047) -> (53.8716, -65.6917)
  line L724 (53.8716, -65.6917) -> (53.9745, -65.8761)
  line L725 (53.9745, -65.8761) -> (54.0822, -66.0577)
  line L726 (54.0822, -66.0577) -> (53.7005, -66.2908)
  line L727 (53.7005, -66.2908) -> (53.6424, -66.3336)
  line L728 (53.6424, -66.3336) -> (53.5871, -66.381)
  line L729 (53.5871, -66.381) -> (53.5337, -66.4313)
  line L730 (53.5337, -66.4313) -> (53.4818, -66.4841)
  line L731 (53.4818, -66.4841) -> (53.4313, -66.5391)
  line L732 (53.4313, -66.5391) -> (53.382, -66.596)
  line L733 (53.382, -66.596) -> (53.334, -66.6547)
  line L734 (53.334, -66.6547) -> (53.2871, -66.7152)
  line L735 (53.2871, -66.7152) -> (53.2414, -66.7772)
  line L736 (53.2414, -66.7772) -> (53.1967, -66.8408)
  line L737 (53.1967, -66.8408) -> (53.1531, -66.9058)
  line L738 (53.1531, -66.9058) -> (53.1105, -66.9723)
  line L739 (53.1105, -66.9723) -> (53.1881, -67.0893)
  line L740 (53.1881, -67.0893) -> (53.2675, -67.2052)
  line L741 (53.2675, -67.2052) -> (53.3485, -67.3199)
  line L742 (53.3485, -67.3199) -> (53.4259, -67.3042)
  line L743 (53.4259, -67.3042) -> (53.5023, -67.2871)
  line L744 (53.5023, -67.2871) -> (53.5777, -67.2684)
  line L745 (53.5777, -67.2684) -> (53.6521, -67.2482)
  line L746 (53.6521, -67.2482) -> (53.7254, -67.2264)
  line L747 (53.7254, -67.2264) -> (53.7975, -67.2028)
  line L748 (53.7975, -67.2028) -> (53.8684, -67.1775)
  line L749 (53.8684, -67.1775) -> (53.9379, -67.1503)
  line L750 (53.9379, -67.1503) -> (54.0059, -67.121)
  line L751 (54.0059, -67.121) -> (54.0722, -67.0894)
  line L752 (54.0722, -67.0894) -> (54.1363, -67.0549)
  line L753 (54.1363, -67.0549) -> (54.1972, -67.0162)
  line L754 (54.1972, -67.0162) -> (54.5526, -66.7447)
  line L755 (54.5526, -66.7447) -> (54.683, -66.9108)
  line L756 (54.683, -66.9108) -> (54.8177, -67.0734)
  line L757 (54.8177, -67.0734) -> (54.9566, -67.2323)
  line L758 (54.9566, -67.2323) -> (55.0997, -67.3876)
  line L759 (55.0997, -67.3876) -> (54.7749, -67.695)
  line L760 (54.7749, -67.695) -> (54.727, -67.749)
  line L761 (54.727, -67.749) -> (54.6827, -67.8068)
  line L762 (54.6827, -67.8068) -> (54.6409, -67.8671)
  line L763 (54.6409, -67.8671) -> (54.6011, -67.9295)
  line L764 (54.6011, -67.9295) -> (54.5631, -67.9938)
  line L765 (54.5631, -67.9938) -> (54.5268, -68.0597)
  line L766 (54.5268, -68.0597) -> (54.492, -68.1271)
  line L767 (54.492, -68.1271) -> (54.4588, -68.196)
  line L768 (54.4588, -68.196) -> (54.4269, -68.2662)
  line L769 (54.4269, -68.2662) -> (54.3964, -68.3377)
  line L770 (54.3964, -68.3377) -> (54.3673, -68.4104)
  line L771 (54.3673, -68.4104) -> (54.3395, -68.4842)
  line L772 (54.3395, -68.4842) -> (54.4397, -68.5826)
  line L773 (54.4397, -68.5826) -> (54.5414, -68.6794)
  line L774 (54.5414, -68.6794) -> (54.6445, -68.7747)
  line L775 (54.6445, -68.7747) -> (54.717, -68.7434)
  line L776 (54.717, -68.7434) -> (54.7881, -68.7107)
  line L777 (54.7881, -68.7107) -> (54.858, -68.6768)
  line L778 (54.858, -68.6768) -> (54.9266, -68.6415)
  line L779 (54.9266, -68.6415) -> (54.9938, -68.6049)
  line L780 (54.9938, -68.6049) -> (55.0594, -68.5669)
  line L781 (55.0594, -68.5669) -> (55.1235, -68.5274)
  line L782 (55.1235, -68.5274) -> (55.1858, -68.4863)
  line L783 (55.1858, -68.4863) -> (55.2462, -68.4435)
  line L784 (55.2462, -68.4435) -> (55.3044, -68.3988)
  line L785 (55.3044, -68.3988) -> (55.36, -68.3518)
  line L786 (55.36, -68.3518) -> (55.4116, -68.3013)
  line L787 (55.4116, -68.3013) -> (55.7028, -67.9618)
  line L788 (55.7028, -67.9618) -> (55.8648, -68.0972)
  line L789 (55.8648, -68.0972) -> (56.0304, -68.2282)
  line L790 (56.0304, -68.2282) -> (56.1993, -68.3548)
  line L791 (56.1993, -68.3548) -> (56.3715, -68.4769)
  line L792 (56.3715, -68.4769) -> (56.1177, -68.8451)
  line L793 (56.1177, -68.8451) -> (56.0821, -68.9079)
  line L794 (56.0821, -68.9079) -> (56.0508, -68.9736)
  line L795 (56.0508, -68.9736) -> (56.0225, -69.0413)
  line L796 (56.0225, -69.0413) -> (55.9965, -69.1107)
  line L797 (55.9965, -69.1107) -> (55.9727, -69.1814)
  line L798 (55.9727, -69.1814) -> (55.9509, -69.2534)
  line L799 (55.9509, -69.2534) -> (55.9309, -69.3266)
  line L800 (55.9309, -69.3266) -> (55.9127, -69.4009)
  line L801 (55.9127, -69.4009) -> (55.8961, -69.4762)
  line L802 (55.8961, -69.4762) -> (55.8812, -69.5524)
  line L803 (55.8812, -69.5524) -> (55.8678, -69.6296)
  line L804 (55.8678, -69.6296) -> (55.8559, -69.7076)
  line L805 (55.8559, -69.7076) -> (55.9744, -69.783)
  line L806 (55.9744, -69.783) -> (56.094, -69.8566)
  line L807 (56.094, -69.8566) -> (56.2147, -69.9284)
  line L808 (56.2147, -69.9284) -> (56.279, -69.8826)
  line L809 (56.279, -69.8826) -> (56.3419, -69.8359)
  line L810 (56.3419, -69.8359) -> (56.4032, -69.7881)
  line L811 (56.4032, -69.7881) -> (56.4629, -69.7394)
  line L812 (56.4629, -69.7394) -> (56.521, -69.6896)
  line L813 (56.521, -69.6896) -> (56.5773, -69.6388)
  line L814 (56.5773, -69.6388) -> (56.6318, -69.5869)
  line L815 (56.6318, -69.5869) -> (56.6842, -69.5337)
  line L816 (56.6842, -69.5337) -> (56.7344, -69.4793)
  line L817 (56.7344, -69.4793) -> (56.782, -69.4235)
  line L818 (56.782, -69.4235) -> (56.8266, -69.3659)
  line L819 (56.8266, -69.3659) -> (56.8666, -69.3058)
  line L820 (56.8666, -69.3058) -> (57.0808, -68.9132)
  line L821 (57.0808, -68.9132) -> (57.2674, -69.0119)
  line L822 (57.2674, -69.0119) -> (57.4566, -69.1056)
  line L823 (57.4566, -69.1056) -> (57.6482, -69.1943)
  line L824 (57.6482, -69.1943) -> (57.8421, -69.2779)
  line L825 (57.8421, -69.2779) -> (57.6703, -69.6909)
  line L826 (57.6703, -69.6909) -> (57.6485, -69.7597)
  line L827 (57.6485, -69.7597) -> (57.6316, -69.8305)
  line L828 (57.6316, -69.8305) -> (57.6179, -69.9026)
  line L829 (57.6179, -69.9026) -> (57.607, -69.9759)
  line L830 (57.607, -69.9759) -> (57.5984, -70.05)
  line L831 (57.5984, -70.05) -> (57.5921, -70.125)
  line L832 (57.5921, -70.125) -> (57.5877, -70.2007)
  line L833 (57.5877, -70.2007) -> (57.5853, -70.2772)
  line L834 (57.5853, -70.2772) -> (57.5848, -70.3543)
  line L835 (57.5848, -70.3543) -> (57.586, -70.432)
  line L836 (57.586, -70.432) -> (57.589, -70.5102)
  line L837 (57.589, -70.5102) -> (57.5936, -70.589)
  line L838 (57.5936, -70.589) -> (57.7252, -70.6381)
  line L839 (57.7252, -70.6381) -> (57.8575, -70.6852)
  line L840 (57.8575, -70.6852) -> (57.9904, -70.7303)
  line L841 (57.9904, -70.7303) -> (58.0438, -70.6722)
  line L842 (58.0438, -70.6722) -> (58.0956, -70.6134)
  line L843 (58.0956, -70.6134) -> (58.1456, -70.554)
  line L844 (58.1456, -70.554) -> (58.1939, -70.4939)
  line L845 (58.1939, -70.4939) -> (58.2404, -70.4331)
  line L846 (58.2404, -70.4331) -> (58.2849, -70.3717)
  line L847 (58.2849, -70.3717) -> (58.3274, -70.3096)
  line L848 (58.3274, -70.3096) -> (58.3676, -70.2467)
  line L849 (58.3676, -70.2467) -> (58.4054, -70.183)
  line L850 (58.4054, -70.183) -> (58.4404, -70.1185)
  line L851 (58.4404, -70.1185) -> (58.472, -70.0529)
  line L852 (58.472, -70.0529) -> (58.4986, -69.9858)
  line L853 (58.4986, -69.9858) -> (58.6265, -69.5573)
  line L854 (58.6265, -69.5573) -> (58.8296, -69.615)
  line L855 (58.8296, -69.615) -> (59.0341, -69.6673)
  line L856 (59.0341, -69.6673) -> (59.24, -69.7143)
  line L857 (59.24, -69.7143) -> (59.447, -69.7558)
  line L858 (59.447, -69.7558) -> (59.3649, -70.1954)
  line L859 (59.3649, -70.1954) -> (59.3578, -70.2672)
  line L860 (59.3578, -70.2672) -> (59.356, -70.34)
  line L861 (59.356, -70.34) -> (59.3577, -70.4134)